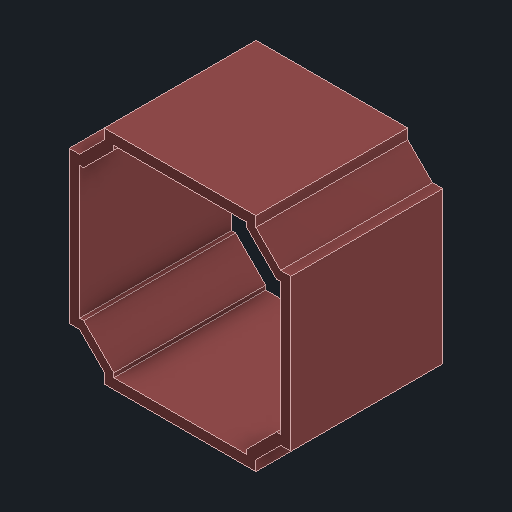
# Autodesk Inventor part: Tunnel Vertical
Saved by Autodesk Inventor 2023.4 (Build 274418000, 418)
## iProperties
Created: 2022-08-10
Part Number: Tunnel Vertical
Material: Generic
Document SubType Name: Modeling
Designer: xSibe
Density: 1 g/cm^3
Appearance: Plastic Brown
Author: xSibe
Autodesk Inventor part; units mm, degrees
ref_plane "YZ Plane" through (0, 0, 0) normal (1, 0, 0) x (0, 1, 0)
ref_plane "XZ Plane" through (0, 0, 0) normal (0, 1, 0) x (-1, 0, 0)
sketch "Sketch1" plane through (0, 0, 0) normal (0, 0, 1) x (1, 0, 0)
  circle A0 centre (-10, 20.9) radius 1.875 projected
  circle A1 centre (-10, -20.9) radius 1.875 projected
  circle A2 centre (10, 20.9) radius 1.875 projected
  circle A3 centre (10, -20.9) radius 1.875 projected
  circle A4 centre (20.8, -14.4) radius 2.075 projected
  circle A5 centre (20.8, 14.4) radius 2.075 projected
  circle A6 centre (-20.8, 14.4) radius 2.075 projected
  circle A7 centre (-20.8, -14.4) radius 2.075 projected
  line L0 (16.9, -16.9) -> (-16.9, -16.9) projected
  line L1 (-16.9, -16.9) -> (-16.9, 16.9) projected
  line L2 (-16.9, 16.9) -> (16.9, 16.9) projected
  line L3 (16.9, 16.9) -> (16.9, -16.9) projected
  line L4 (-17.05, 24.9) -> (-17.05, 22.55) projected
  line L5 (-17.05, 22.55) -> (-22.55, 17.05) projected
  line L6 (-22.55, 17.05) -> (-24.9, 17.05) projected
  line L7 (-24.9, 17.05) -> (-24.9, -17.05) projected
  line L8 (-24.9, -17.05) -> (-22.55, -17.05) projected
  line L9 (-22.55, -17.05) -> (-17.05, -22.55) projected
  line L10 (-17.05, -22.55) -> (-17.05, -24.9) projected
  line L11 (-17.05, -24.9) -> (17.05, -24.9) projected
  line L12 (17.05, -24.9) -> (17.05, -22.55) projected
  line L13 (17.05, -22.55) -> (22.55, -17.05) projected
  line L14 (22.55, -17.05) -> (24.9, -17.05) projected
  line L15 (24.9, -17.05) -> (24.9, 17.05) projected
  line L16 (24.9, 17.05) -> (22.55, 17.05) projected
  line L17 (22.55, 17.05) -> (17.05, 22.55) projected
  line L18 (17.05, 22.55) -> (17.05, 24.9) projected
  line L19 (17.05, 24.9) -> (-17.05, 24.9) projected
  line L20 (24.825, 16.975) -> (24.825, -16.975)
  line L21 (24.825, -16.975) -> (22.5189, -16.975)
  line L22 (22.5189, -16.975) -> (16.975, -22.5189)
  line L23 (16.975, -22.5189) -> (16.975, -24.825)
  line L24 (16.975, -24.825) -> (-16.975, -24.825)
  line L25 (-16.975, -24.825) -> (-16.975, -22.5189)
  line L26 (-16.975, -22.5189) -> (-22.5189, -16.975)
  line L27 (-22.5189, -16.975) -> (-24.825, -16.975)
  line L28 (-24.825, -16.975) -> (-24.825, 16.975)
  line L29 (-24.825, 16.975) -> (-22.5189, 16.975)
  line L30 (-22.5189, 16.975) -> (-16.975, 22.5189)
  line L31 (-16.975, 22.5189) -> (-16.975, 24.825)
  line L32 (-16.975, 24.825) -> (16.975, 24.825)
  line L33 (16.975, 24.825) -> (16.975, 22.5189)
  line L34 (16.975, 22.5189) -> (22.5189, 16.975)
  line L35 (22.5189, 16.975) -> (24.825, 16.975)
  line L36 (22.5189, -16.975) -> (22.5189, 16.975)
  line L37 (16.975, 22.5189) -> (-16.975, 22.5189)
  line L38 (-22.5189, 16.975) -> (-22.5189, -16.975)
  line L39 (-16.975, -22.5189) -> (16.975, -22.5189)
  line L40 (16.975, 24.825) -> (24.825, 24.825)
  line L41 (24.825, 24.825) -> (24.825, 16.975)
  line L42 (24.825, 24.825) -> (14.825, 24.825)
  line L43 (14.825, 24.825) -> (14.825, 21.575)
  line L44 (21.575, 14.825) -> (24.825, 14.825)
  line L45 (24.825, 14.825) -> (24.825, 24.825)
  line L46 (14.825, 21.575) -> (21.575, 14.825)
  line L47 (-21.575, 14.825) -> (-14.825, 21.575)
  line L48 (-14.825, 21.575) -> (-14.825, 24.825)
  line L49 (-24.825, 14.825) -> (-21.575, 14.825)
  line L50 (-14.825, -21.575) -> (-21.575, -14.825)
  line L51 (-21.575, -14.825) -> (-24.825, -14.825)
  line L52 (-14.825, -24.825) -> (-14.825, -21.575)
  line L53 (21.575, -14.825) -> (14.825, -21.575)
  line L54 (14.825, -21.575) -> (14.825, -24.825)
  line L55 (24.825, -14.825) -> (21.575, -14.825)
  point P0 (0, 0)
  point P1 (14.825, 14.825)
  point P2 (22.5189, 14.825)
  point P3 (22.5189, -14.825)
  point P4 (14.825, -22.5189)
  point P5 (-14.825, -22.5189)
  point P6 (-22.5189, -14.825)
  point P7 (-22.5189, 14.825)
  point P8 (-14.825, 22.5189)
  point P9 (14.825, 22.5189)
  dimension "d0" = 0.075
  dimension "d3" = 360
  dimension "d5" = 10
  dimension "d6" = 10
  dimension "d7" = 6.75
  dimension "d8" = 6.75
  dimension "d11" = 360
  constraints: 72 end point, 2 horizontal, 2 parallel, 2 perpendicular, 2 point on line, 1 collinear, 57 other
  measures "d0" distance between parallel lines of L15 L20
  measures "d5" distance of L44.end point (14.825, 14.825)
  measures "d6" distance of point (14.825, 14.825) L42.end
  measures "d7" distance of L43.end point (14.825, 14.825)
  measures "d8" distance of L44.start point (14.825, 14.825)
ref_plane "Work Plane1" through (-24.9, -24.9, 7.7) normal (0, 0, 1) x (1, 0, 0)
extrude "Extrusion1" add sketch "Sketch1" along normal blind 34 from surface at 7.7 contours L37 A0 | A0 L37 L48 L32 L43 A2 | A2 L37 | L48 L47 A6 L38 L30 L37 | L37 L31 L32 L48 | L43 L32 L33 L37 | L37 L34 L36 A5 L46 L43 | L38 A6 L49 L28 L29 | L47 L49 L38 A6 | L38 L49 A6 | L35 L20 L44 A5 L36 | A5 L36 L44 L46 | L49 A6 L38 A7 L51 L28 | L49 L38 A6 | A5 L44 L36 | L36 L44 A5 | A5 L44 L20 L55 A4 L36 | L51 A7 L38 L27 L28 | L38 L51 A7 | A4 L55 L36 | L51 L38 A7 | L51 L50 A7 L38 | L20 L21 L36 A4 L55 | L53 L55 L36 A4 | A4 L36 L22 L39 L54 L53 | L55 A4 L36 | L38 A7 L50 L52 L39 L26 | L39 L52 L24 L25 | L54 L24 L52 L39 A1 A3 | L39 L23 L24 L54 | A3 L39 | L39 A1 picked at (-9.805, 22.5731) picked at (9.805, 22.5731) picked at (-20.715, 15.8728) picked at (20.715, 15.8728) picked at (-20.715, -15.8728) picked at (20.715, -15.8728) picked at (10.195, -22.5731) picked at (-9.805, -22.5731)
body "Solid1"
